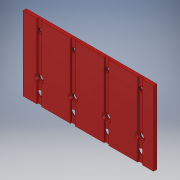
# Autodesk Inventor part: talon stack zip tie mount
Saved by Autodesk Inventor 2019 (Build 230136000, 136)
## iProperties
Created: 2019-01-16
Part Number: talon stack zip tie mount
Material: ABS Plastic
Document SubType Name: Modeling
Designer: pctech
Density: 1.06 g/cm^3
Appearance: Red
Mass: 31.6682 g
Surface Area: 185.044 cm^2
Volume: 26.3901 cm^3
Author: pctech
Autodesk Inventor part; units mm, degrees
ref_plane "YZ Plane" through (0, 0, 0) normal (1, 0, 0) x (0, 1, 0)
ref_plane "XZ Plane" through (0, 0, 0) normal (0, 1, 0) x (-1, 0, 0)
ref_plane "XY Plane" through (0, 0, 0) normal (0, 0, 1) x (1, 0, 0)
sketch "Sketch1" plane through (0, 0, 0) normal (0, 0, 1) x (1, 0, 0)
  line L0 (0, 0) -> (123.19, 0)
  line L1 (123.19, 0) -> (123.19, 69.85)
  line L2 (123.19, 69.85) -> (0, 69.85)
  line L3 (0, 69.85) -> (0, 0)
  dimension "d0" = 69.85
  dimension "d1" = 123.19
  constraints: 8 end point, 2 parallel, 1 horizontal, 1 perpendicular
  measures "d0" distance of L2.end L0.start
  measures "d1" distance of L0.start L0.end
extrude "Extrusion1" add sketch "Sketch1" along normal blind 3.175
sketch "Sketch2" plane through (0, 0, 3.175) normal (0, 0, 1) x (1, 0, 0)
  line L0 (123.19, 69.85) -> (0, 69.85) projected
  line L1 (0, 69.85) -> (0, 0) projected
  point P0 (15.24, 60.071)
  point P1 (46.99, 60.071)
  point P2 (78.74, 60.071)
  point P3 (110.49, 60.071)
  dimension "d5" = 9.779
  dimension "d6" = 15.24
  dimension "d7" = 31.75
  dimension "d8" = 31.75
  dimension "d9" = 31.75
  constraints: 3 horizontal alignment
  measures "d5" distance from line of L0 point (15.24, 60.071)
  measures "d6" distance from line of L1 point (15.24, 60.071)
  measures "d7" distance of point (46.99, 60.071) point (15.24, 60.071)
  measures "d8" distance of point (78.74, 60.071) point (46.99, 60.071)
  measures "d9" distance of point (110.49, 60.071) point (78.74, 60.071)
hole "Hole1" at (15.24, 60.071, 3.175) at (46.99, 60.071, 3.175) at (78.74, 60.071, 3.175) at (110.49, 60.071, 3.175) direction (0, 0, -1) diameter 4.4958 end through all clearance for "Flat Head Machine Screw (82)" size "#8" standard "Ansi Unified Screw Threads"
sketch "Sketch3" plane through (0, 0, 3.175) normal (0, 0, 1) x (1, 0, 0)
  circle A0 centre (110.49, 60.071) radius 2.2479 projected
  circle A1 centre (46.99, 60.071) radius 2.2479 projected
  circle A2 centre (15.24, 60.071) radius 2.2479 projected
  circle A3 centre (78.74, 60.071) radius 2.2479 projected
  line L0 (0, 0) -> (123.19, 0) projected
  line L1 (123.19, 0) -> (123.19, 69.85) projected
  line L2 (123.19, 69.85) -> (0, 69.85) projected
  line L3 (0, 69.85) -> (0, 0) projected
  point P0 (15.24, 21.5392)
  point P1 (46.99, 21.5392)
  point P2 (78.74, 21.5392)
  point P3 (110.49, 21.5392)
  constraints: 3 horizontal alignment
hole "Hole2" at (15.24, 21.5392, 3.175) at (46.99, 21.5392, 3.175) at (78.74, 21.5392, 3.175) at (110.49, 21.5392, 3.175) direction (0, 0, -1) diameter 4.4958 end through all countersink diameter 8.4328 countersink angle 82 clearance for "Flat Head Machine Screw (82)" size "#8" standard "Ansi Unified Screw Threads"
sketch "Sketch4" plane through (0, 0, 0) normal (0, 0, -1) x (-1, 0, 0)
  circle A0 centre (-78.74, 21.5392) radius 2.2479 projected
  circle A1 centre (-15.24, 21.5392) radius 2.2479 projected
  circle A2 centre (-46.99, 21.5392) radius 2.2479 projected
  circle A3 centre (-110.49, 21.5392) radius 2.2479 projected
  circle A4 centre (-78.74, 60.071) radius 2.2479 projected
  circle A5 centre (-15.24, 60.071) radius 2.2479 projected
  circle A6 centre (-46.99, 60.071) radius 2.2479 projected
  circle A7 centre (-110.49, 60.071) radius 2.2479 projected
  line L0 (0, 0) -> (-123.19, 0) projected
  line L1 (0, 69.85) -> (0, 0) projected
  line L2 (-123.19, 69.85) -> (0, 69.85) projected
  line L3 (-123.19, 0) -> (-123.19, 69.85) projected
  point P0 (-110.49, 9.271)
  point P1 (-78.74, 9.271)
  point P2 (-46.99, 9.271)
  point P3 (-15.24, 9.271)
  dimension "d26" = 50.8
  constraints: 4 vertical alignment, 3 horizontal alignment
  measures "d26" distance of A5.centre point (-15.24, 9.271)
hole "Hole3" at (110.49, 9.271, 0) at (78.74, 9.271, 0) at (46.99, 9.271, 0) at (15.24, 9.271, 0) direction (0, 0, 1) diameter 4.4958 end through all countersink diameter 8.4328 countersink angle 82 clearance for "Flat Head Machine Screw (82)" size "#8" standard "Ansi Unified Screw Threads"
sketch "Sketch5" plane through (0, 0, 3.175) normal (0, 0, 1) x (1, 0, 0)
  circle A0 centre (46.99, 9.271) radius 2.2479 construction
  circle A1 centre (110.49, 9.271) radius 2.2479 construction
  circle A2 centre (78.74, 9.271) radius 2.2479 construction
  circle A3 centre (15.24, 9.271) radius 2.2479 construction
  circle A4 centre (78.74, 21.5392) radius 4.2164 construction
  circle A5 centre (15.24, 21.5392) radius 4.2164 construction
  circle A6 centre (46.99, 21.5392) radius 4.2164 construction
  circle A7 centre (110.49, 21.5392) radius 4.2164 construction
  circle A8 centre (78.74, 60.071) radius 2.2479 construction
  circle A9 centre (15.24, 60.071) radius 2.2479 construction
  circle A10 centre (46.99, 60.071) radius 2.2479 construction
  circle A11 centre (110.49, 60.071) radius 2.2479 construction
  line L0 (0, 0) -> (123.19, 0) construction
  line L1 (123.19, 0) -> (123.19, 69.85) construction
  line L2 (123.19, 69.85) -> (0, 69.85) construction
  line L3 (0, 69.85) -> (0, 0) construction
  circle A12 centre (15.24, 21.5392) radius 2.2479 projected
  line L4 (12.9921, 69.85) -> (12.9921, 0)
  line L5 (17.4879, 69.85) -> (17.4879, 0)
  line L6 (12.9921, 69.85) -> (17.4879, 69.85)
  line L7 (12.9921, 0) -> (17.4879, 0)
  line L8 (0, 0) -> (123.19, 0) projected
  circle A13 centre (15.24, 60.071) radius 2.2479 projected
  constraints: 8 end point, 4 point on line, 2 perpendicular, 2 tangent, 1 coincident, 1 collinear, 1 horizontal
extrude "Extrusion2" cut sketch "Sketch5" against normal blind 1.27 contours L5 L7 L4 A12 | A12 L4 A13 L5 | A13 L4 L6 L5
pattern_linear "Rectangular Pattern1" count 4 spacing 31.75 along (1, 0, 0) of "Extrusion2"
equation "\"d8\" = d7"
equation "\"d9\" = d7"
body "Solid1"
